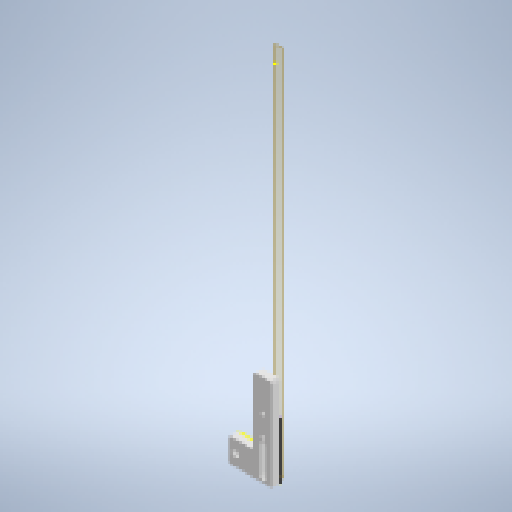
# Autodesk Inventor part: крепление ремня
Saved by Autodesk Inventor 2024.2 (Build 282272000, 272)
## iProperties
Created: 2026-02-20
Part Number: крепление ремня
Material: Типовые
Document SubType Name: Modeling
Designer: katya_notebook
Density: 1 g/cm^3
Appearance: По умолчанию
Author: katya_notebook
Autodesk Inventor part; units mm, degrees
ref_plane "YZ Plane" through (0, 0, 0) normal (1, 0, 0) x (0, 1, 0)
ref_plane "XZ Plane" through (0, 0, 0) normal (0, 1, 0) x (-1, 0, 0)
ref_plane "XY Plane" through (0, 0, 0) normal (0, 0, 1) x (1, 0, 0)
ref_plane "РабПлоскость1" through (0, 0, 0) normal (0, 0, 1) x (1, 0, 0)
sketch "Эскиз1" plane through (0, 0, 0) normal (0, 0, 1) x (1, 0, 0)
  line L0 (-10.3, -267.007) -> (3.7, -267.007)
  line L1 (-26.3, -267.007) -> (-10.3, -267.007) projected
  arc A0 (-28.3, -265.007) -> (-26.3, -267.007) centre (-26.3, -265.007) ccw projected
  line L2 (-28.3, -251.007) -> (-28.3, -265.007) projected
  arc A1 (-26.3, -249.007) -> (-28.3, -251.007) centre (-26.3, -251.007) ccw projected
  line L3 (-10.3, -249.007) -> (-26.3, -249.007) projected
  line L4 (-10.3, -201.4771) -> (-10.3, -249.007) projected
  arc A2 (-8.3, -199.4771) -> (-10.3, -201.4771) centre (-8.3, -201.4771) ccw projected
  line L5 (1.7, -199.4771) -> (-8.3, -199.4771) projected
  arc A3 (3.7, -201.4771) -> (1.7, -199.4771) centre (1.7, -201.4771) ccw projected
  line L6 (3.7, -267.007) -> (3.7, -201.4771) projected
  line L7 (3.7, -267.007) -> (-10.3, -267.007)
  line L8 (-1.0506, -258.007) -> (-1.0506, -243.007)
  line L9 (-5.5498, -258.007) -> (-5.5498, -243.007)
  arc A4 (-1.0506, -243.007) -> (-5.5498, -243.007) centre (-3.3002, -243.007) ccw
  arc A5 (-5.5498, -263.1742) -> (-1.0506, -263.1742) centre (-3.3002, -263.2319) ccw
  line L10 (-5.5498, -263.2896) -> (-5.5498, -258.007)
  line L11 (-1.0506, -263.2896) -> (-1.0506, -258.007)
  circle A6 centre (-23.3, -258.4837) radius 2.25 projected
  circle A7 centre (-3.3, -238.0001) radius 1.25 projected
  circle A8 centre (-3.3, -223.0001) radius 1.25 projected
  point P0 (0, 0)
  dimension "d2" = 15
  constraints: 12 end point, 6 point on circle, 3 vertical, 2 centre point, 2 equal length, 2 point on line, 2 tangent, 1 horizontal
  measures "d2" distance of L9.start L9.end
extrude "Выдавливание1" add sketch "Эскиз1" along normal blind 6
sketch "Эскиз2" plane through (0, 0, 0) normal (0, 0, -1) x (-1, 0, 0)
  line L0 (10.3, -225.242) -> (-3.7, -225.242)
  circle A0 centre (3.3, -238.0001) radius 1.25 projected
  circle A1 centre (3.3, -229.8361) radius 1.25
  line L1 (26.3, -267.007) -> (-3.7, -267.007) projected
  arc A2 (26.3, -267.007) -> (28.3, -265.007) centre (26.3, -265.007) ccw projected
  line L2 (28.3, -251.007) -> (28.3, -265.007) projected
  arc A3 (28.3, -251.007) -> (26.3, -249.007) centre (26.3, -251.007) ccw projected
  line L3 (10.3, -249.007) -> (26.3, -249.007) projected
  circle A4 centre (23.3, -258.4837) radius 2.25 projected
  line L4 (1.0506, -243.007) -> (1.0506, -263.1742) projected
  arc A5 (5.5498, -243.007) -> (1.0506, -243.007) centre (3.3002, -243.007) ccw projected
  line L5 (5.5498, -263.1742) -> (5.5498, -243.007) projected
  arc A6 (1.0506, -263.1742) -> (5.5498, -263.1742) centre (3.3002, -263.2319) ccw projected
  line L6 (-3.7, -225.242) -> (-3.7, -267.007)
  line L7 (10.3, -249.007) -> (10.3, -225.242)
  point P0 (0, 0)
  constraints: 6 end point, 1 centre point, 1 equal radius, 1 horizontal, 1 parallel, 1 vertical
